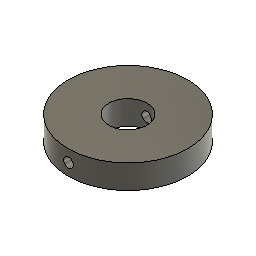
Small Compactor (Autodesk Fusion 360 design; units mm, degrees)
Autodesk Fusion 360 part; units mm, degrees
sketch "Eskiz1" plane through (0, 0, 0) normal (0, 1, 0) x (1, 0, 0)
  circle A0 centre (0, 0) radius 12.5
  circle A1 centre (0, 0) radius 4
  dimension "d1" = 25
  dimension "d2" = 8
  constraint coincident A0.centre A1.centre
  measures "d1" diameter of A0
  measures "d2" diameter of A1
extrude "Ekstrüde Et1" add sketch "Eskiz1" along normal blind 5
sketch "Eskiz2" plane through (0, 0, 0) normal (0, 0, 1) x (1, 0, 0)
  circle A0 centre (0, 2.5) radius 1
  dimension "d5" = 2
  dimension "d6" = 2.5
  measures "d5" diameter of A0
  measures "d6" distance of origin A0.centre
extrude "Ekstrüde Et2" cut sketch "Eskiz2" along normal blind 17 and the other way blind 18
